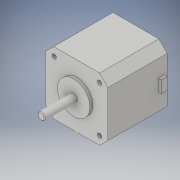
# Autodesk Inventor part: Motor BYGHW609
Saved by Autodesk Inventor 2019 (Build 230136000, 136)
## iProperties
Created: 2018-12-23
Part Number: Motor BYGHW609
Material: Generic
Document SubType Name: Modeling
Designer: Martin
Density: 1 g/cm^3
Appearance: Default
Author: Martin
Autodesk Inventor part; units mm, degrees
ref_plane "YZ Plane" through (0, 0, 0) normal (1, 0, 0) x (0, 1, 0)
ref_plane "XZ Plane" through (0, 0, 0) normal (0, 1, 0) x (-1, 0, 0)
ref_plane "XY Plane" through (0, 0, 0) normal (0, 0, 1) x (1, 0, 0)
sketch "Sketch1" plane through (0, 0, 0) normal (0, 0, 1) x (1, 0, 0)
  line L0 (15.5, -21.15) -> (-15.5, -21.15)
  line L1 (-21.15, -15.5) -> (-21.15, 15.5)
  line L2 (-15.5, 21.15) -> (15.5, 21.15)
  line L3 (21.15, 15.5) -> (21.15, -15.5)
  line L4 (21.15, -21.15) -> (-21.15, 21.15) construction
  line L5 (-21.15, -21.15) -> (21.15, 21.15) construction
  line L6 (-15.5, 21.15) -> (-21.15, 15.5)
  line L7 (-21.15, 0) -> (-21.15, 15.5)
  line L8 (0, 21.15) -> (-15.5, 21.15)
  line L9 (15.5, 21.15) -> (21.15, 15.5)
  line L10 (21.15, -15.5) -> (15.5, -21.15)
  line L11 (-15.5, -21.15) -> (-21.15, -15.5)
  point P0 (0, 0)
  dimension "d0" = 42.3
  dimension "d1" = 42.3
  dimension "d2" = 5.65
  dimension "d3" = 5.65
  dimension "d4" = 15.5
  dimension "d5" = 15.5
  constraints: 24 end point, 10 point on line, 4 midpoint, 2 parallel, 1 horizontal, 1 perpendicular
  measures "d0" distance of L4.end L5.end
  measures "d1" distance of L5.start L4.end
  measures "d2" distance of L2.start L4.end
  measures "d3" distance of L1.end L4.end
  measures "d4" distance of L7.start L7.end
  measures "d5" distance of L8.start L8.end
extrude "Extrusion1" add sketch "Sketch1" against normal blind 40
sketch "Sketch2" plane through (0, 0, 0) normal (0, 0, 1) x (1, 0, 0)
  circle A0 centre (0, 0) radius 11
  dimension "d8" = 22
  constraints: 1 centre point, 1 coincident
  measures "d8" diameter of A0
extrude "Extrusion2" add sketch "Sketch2" along normal blind 2
sketch "Sketch3" plane through (0, 0, 0) normal (0, 0, 1) x (1, 0, 0)
  circle A0 centre (0, 0) radius 2.5
  dimension "d11" = 5
  constraints: 1 centre point, 1 coincident
  measures "d11" diameter of A0
extrude "Extrusion3" add sketch "Sketch3" along normal blind 24
chamfer "Chamfer1" distance 0.5 angle 45 1 edges at (-2.5, 0, 24)
sketch "Sketch4" plane through (0, 0, 0) normal (0, 0, 1) x (1, 0, 0)
  line L0 (-21.15, 15.5) -> (-21.15, -15.5) projected
  line L1 (-15.5, 21.15) -> (-21.15, 15.5) projected
  circle A0 centre (-15.1766, 15.5) radius 1.5
  circle A1 centre (15.5, 15.5) radius 1.5
  circle A2 centre (-15.5, -15.5) radius 1.5
  circle A3 centre (15.5, -15.5) radius 1.5
  point P0 (0, 0)
  dimension "d18" = 3
  dimension "d19" = 3
  dimension "d20" = 3
  dimension "d21" = 3
  constraints: 4 centre point
  measures "d18" diameter of A0
  measures "d19" diameter of A1
  measures "d20" diameter of A2
  measures "d21" diameter of A3
extrude "Extrusion4" cut sketch "Sketch4" against normal blind 4.5
sketch "Sketch5" plane through (-15.5, -21.15, 0) normal (0, -1, 0) x (1, 0, 0)
  point P0 (15.5, 0)
sketch "Sketch6" plane through (21.15, -15.5, 0) normal (1, 0, 0) x (0, 0, -1)
  line L0 (40, 0) -> (40, 31) projected
  line L1 (38, 11.5) -> (34, 11.5)
  line L2 (34, 11.5) -> (34, 19.5)
  line L3 (34, 19.5) -> (38, 19.5)
  line L4 (38, 19.5) -> (38, 11.5)
  line L5 (38, 11.5) -> (34, 19.5) construction
  line L6 (34, 11.5) -> (38, 19.5) construction
  line L7 (0, 0) -> (40, 0) projected
  line L8 (0, 31) -> (40, 31) projected
  point P0 (0, 15.5)
  point P1 (40, 15.5)
  point P2 (36, 15.5)
  dimension "d24" = 4
  dimension "d25" = 8
  dimension "d26" = 2
  dimension "d29" = 15.5
  dimension "d30" = 31
  constraints: 12 end point, 3 midpoint, 2 parallel, 1 horizontal, 1 perpendicular
  measures "d24" distance of L2.end L3.end
  measures "d25" distance of L1.end L2.end
  measures "d26" distance between parallel lines of L0 L4
  measures "d29" distance from line of L7 point (36, 15.5)
  measures "d30" distance between parallel lines of L7 L8
extrude "Extrusion5" add sketch "Sketch6" along normal blind 2
equation "\"d3\" = d2"
equation "\"d29\" = 0.5 * d30"
body "Solid1"
